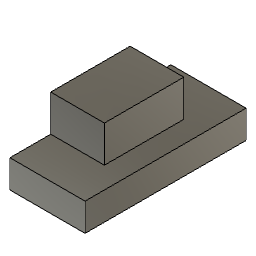
72pin Insert v1 (Autodesk Fusion 360 design; units mm, degrees)
Autodesk Fusion 360 part; units mm, degrees
sketch "Sketch1" plane through (0, 0, 0) normal (0, 0, 1) x (1, 0, 0)
  line L0 (0, 0) -> (3.5, 0)
  line L1 (3.5, 0) -> (3.5, 7.5)
  line L2 (3.5, 7.5) -> (0, 7.5)
  line L3 (0, 7.5) -> (0, 0)
  dimension "d1" = 7.5
  dimension "d2" = 3.5
  constraint horizontal L0
  constraint vertical L1
  constraint horizontal L2
  constraint vertical L3
  constraint coincident L0.start L3.end
  measures "d1" distance of L0.start L2.end
  measures "d2" distance of L1.end L2.end
extrude "Extrude1" add sketch "Sketch1" along normal blind 1.3
sketch "Sketch2" plane through (0, 0, 0) normal (0, 0, 1) x (1, 0, 0)
  line L0 (0, 5.6) -> (2.5, 5.6)
  line L1 (2.5, 5.6) -> (2.5, 1.9)
  line L2 (2.5, 1.9) -> (0, 1.9)
  line L3 (0, 1.9) -> (0, 5.6)
  dimension "d5" = 2.5
  dimension "d6" = 3.7
  dimension "d7" = 1.9
  constraint horizontal L0
  constraint vertical L1
  constraint horizontal L2
  constraint vertical L3
  measures "d5" distance of L0.start L0.end
  measures "d6" distance of L0.start L2.end
  measures "d7" distance of origin L2.end
extrude "Extrude2" add sketch "Sketch2" along normal blind 3
